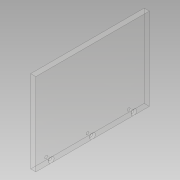
# Autodesk Inventor part: LATERAL A
Saved by Autodesk Inventor 2019 (Build 230136000, 136)
## iProperties
Created: 2020-04-08
Part Number: LATERAL A
Material: Plástico PMMA
Document SubType Name: Modeling
Designer: Luis Pujol
Density: 1.188 g/cm^3
Appearance: Policarbonato - Claro
Author: Luis Pujol
Autodesk Inventor part; units mm, degrees
ref_plane "YZ Plane" through (0, 0, 0) normal (1, 0, 0) x (0, 1, 0)
ref_plane "XZ Plane" through (0, 0, 0) normal (0, 1, 0) x (-1, 0, 0)
ref_plane "XY Plane" through (0, 0, 0) normal (0, 0, 1) x (1, 0, 0)
sketch "Boceto1" plane through (0, 0, 0) normal (1, 0, 0) x (0, 1, 0)
  line L0 (-80, 110) -> (80, 110)
  line L1 (80, 110) -> (80, -110)
  line L2 (80, -110) -> (-80, -110)
  line L3 (-80, -110) -> (-80, 110)
  line L4 (-80, 110) -> (80, -110) construction
  line L5 (80, 110) -> (-80, -110) construction
  point P0 (0, 0)
  dimension "d0" = 160
  dimension "d1" = 220
  constraints: 12 end point, 2 midpoint, 2 parallel, 1 horizontal, 1 perpendicular
  measures "d0" distance of L1.end L2.end
  measures "d1" distance of L0.end L1.end
extrude "Extrusión1" add sketch "Boceto1" along normal blind 10
sketch "Boceto2" plane through (10, 0, 0) normal (1, 0, 0) x (0, 0, -1)
  line L0 (-109, 0) -> (109, 0) construction
  line L1 (110, 80) -> (-110, 80) construction
  line L2 (-110, 80) -> (-110, -80) construction
  line L3 (110, -80) -> (110, 80) construction
  point P0 (0, 0)
  point P1 (0, -75)
  point P2 (80, -75)
  point P3 (-80, -75)
  constraints: 2 end point, 2 horizontal
hole "Agujero1" at (10, -75, 80) at (10, -75, 0) at (10, -75, -80) direction (-1, 0, 0) diameter 5.5 depth 20 tip angle 118 countersink diameter 11 countersink angle 90
